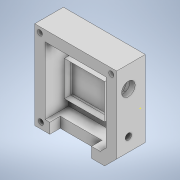
# Autodesk Inventor part: AmpClipOn
Saved by Autodesk Inventor 2020 (Build 240168000, 168)
## iProperties
Created: 2019-05-29
Part Number: AmpClipOn
Material: Generic
Document SubType Name: Modeling
Designer: Dammy
Density: 1 g/cm^3
Appearance: Default
Author: Dammy
Autodesk Inventor part; units mm, degrees
ref_plane "YZ Plane" through (0, 0, 0) normal (1, 0, 0) x (0, 1, 0)
ref_plane "XZ Plane" through (0, 0, 0) normal (0, 1, 0) x (-1, 0, 0)
ref_plane "XY Plane" through (0, 0, 0) normal (0, 0, 1) x (1, 0, 0)
sketch "Sketch1" plane through (0, 0, 0) normal (0, 0, 1) x (1, 0, 0)
  line L0 (11.825, -16.125) -> (-11.825, -16.125)
  line L1 (-14.625, -13.325) -> (-14.625, 16.125)
  line L2 (-14.625, 16.125) -> (14.625, 16.125)
  line L3 (14.625, 16.125) -> (14.625, -13.325)
  line L4 (14.625, -16.125) -> (-14.625, 16.125) construction
  line L5 (-14.625, -16.125) -> (14.625, 16.125) construction
  line L6 (11.825, -16.125) -> (14.625, -13.325)
  line L7 (-14.625, -13.325) -> (-14.625, -16.125)
  line L8 (-11.825, -16.125) -> (-14.625, -16.125)
  point P0 (0, 0)
  dimension "d0" = 29.25
  dimension "d1" = 32.25
  dimension "d56" = 2.8
  dimension "d57" = 2.8
  constraints: 18 end point, 4 point on line, 2 midpoint, 2 parallel, 2 perpendicular, 1 horizontal, 1 vertical
  measures "d0" distance of L1.end L2.end
  measures "d1" distance of L5.start L1.end
  measures "d56" distance of L0.start L4.start
  measures "d57" distance of L3.end L4.start
extrude "Extrusion1" add sketch "Sketch1" along normal blind 11.25
shell "Shell2" thickness 5 outward yes removed faces 1 at (-4.875, -3.5083, 11.25)
sketch "Sketch3" plane through (0, 0, 11.25) normal (0, 0, 1) x (1, 0, 0)
  line L0 (19.625, 21.125) -> (-19.625, 21.125) construction
  line L1 (-14.625, 16.125) -> (14.625, 16.125) construction
  line L2 (-19.625, 21.125) -> (-14.625, 16.125) construction
  line L3 (14.625, 16.125) -> (19.625, 21.125) construction
  line L4 (11.825, -16.125) -> (-14.625, -16.125) construction
  circle A0 centre (-17.125, 18.625) radius 1.25
  circle A1 centre (17.125, 18.625) radius 1.25
  line L5 (-14.625, -16.125) -> (-14.625, 16.125) construction
  line L6 (-14.625, -16.125) -> (-18.625, -20.125) construction
  circle A2 centre (-16.625, -18.125) radius 1.25
  point P0 (0, 0)
  point P1 (18.625, -20.125)
  point P2 (14.625, -16.125)
  point P3 (-11.825, -16.125)
  dimension "d14" = 2.5
  dimension "d15" = 2.5
  dimension "d58" = 2.5
  constraints: 6 end point, 3 centre point, 3 midpoint
  measures "d14" diameter of A0
  measures "d15" diameter of A1
  measures "d58" diameter of A2
extrude "Extrusion3" cut sketch "Sketch3" against normal through all
sketch "Sketch11" plane through (0, 0, 11.25) normal (0, 0, 1) x (1, 0, 0)
  line L0 (-19.625, -21.125) -> (13.8961, -21.125) projected
  line L1 (-14.625, -16.125) -> (11.825, -16.125) projected
  line L2 (7.625, -21.125) -> (-12.375, -21.125)
  line L3 (-12.375, -21.125) -> (-12.375, -16.125)
  line L4 (-12.375, -16.125) -> (7.625, -16.125)
  line L5 (7.625, -16.125) -> (7.625, -21.125)
  circle A0 centre (-16.625, -18.125) radius 1.25 projected
  line L6 (-19.625, 21.125) -> (-19.625, -21.125) projected
  point P0 (0, 0)
  point P1 (-13.4819, -20.125)
  point P2 (18.625, -20.125)
  point P3 (-11.825, -16.125)
  point P4 (14.625, -16.125)
  point P5 (13.8961, -21.125)
  point P6 (7.625, -16.125)
  dimension "d60" = 20
  dimension "d87" = 7.25
  constraints: 8 end point, 2 parallel, 1 horizontal, 1 perpendicular, 1 point on line, 2 other
  measures "d60" distance between parallel lines of L5 L3
  measures "d87" distance between parallel lines of L6 L3
extrude "Extrusion11" cut sketch "Sketch11" against normal blind 5 contours L3 L1 L5 L0
sketch "Sketch13" plane through (19.625, -15.3961, -5) normal (1, 0, 0) x (0, 0, -1)
  line L0 (-11.5, 18.8569) -> (-11.5, 3.8569) construction
  circle A0 centre (-10.625, 26.2711) radius 3.25
  line L1 (-16.25, 0) -> (-16.25, 36.5211) construction
  line L2 (0, 0) -> (-16.25, 0) construction
  line L3 (0, 36.5211) -> (-16.25, 36.5211) projected
  line L4 (-5, 2.0711) -> (-5, 31.5211) projected
  point P0 (-5, 15.3961)
  dimension "d61" = 6.5
  dimension "d81" = 10.25
  dimension "d86" = 5.625
  constraints: 1 centre point
  measures "d61" diameter of A0
  measures "d81" distance from line of L3 A0.centre
  measures "d86" distance from line of A0.centre L4
extrude "Extrusion13" cut sketch "Sketch13" against normal up to surface (5 mm away)
sketch "Sketch14" plane through (-14.625, 16.125, 0) normal (0, 0, 1) x (1, 0, 0)
  line L0 (2, -11.5) -> (19.25, -11.5)
  line L1 (19.25, -11.5) -> (19.25, -26.25)
  line L2 (19.25, -26.25) -> (2, -26.25)
  line L3 (2, -26.25) -> (2, -11.5)
  line L4 (1.25, -10.5) -> (20, -10.5)
  line L5 (20.25, -11.25) -> (20.25, -27)
  line L6 (19.45, -27.25) -> (1.25, -27.25)
  line L7 (1, -27) -> (1, -10.75)
  line L8 (0, -32.25) -> (0, 0) projected
  line L9 (2.25, -32.25) -> (0, -32.25) projected
  line L10 (20, -10.5) -> (20.25, -10.5)
  line L11 (20.25, -10.5) -> (20.25, -11.25)
  line L12 (19.45, -27.25) -> (20.25, -27.25)
  line L13 (20.25, -27.25) -> (20.25, -27)
  line L14 (1.25, -27.25) -> (1, -27.25)
  line L15 (1, -27) -> (1, -27.25)
  line L16 (1, -10.75) -> (1, -10.5)
  line L17 (1.25, -10.5) -> (1, -10.5)
  point P0 (14.625, -16.125)
  point P1 (10.625, -11.5)
  point P2 (10.625, -10.5)
  point P3 (1, -18.875)
  point P4 (2, -18.875)
  dimension "d66" = 1
  dimension "d67" = 1
  dimension "d69" = 17.25
  dimension "d70" = 14.75
  dimension "d71" = 1
  dimension "d72" = 5
  dimension "d83" = 1
  dimension "d84" = 1
  constraints: 32 end point, 7 perpendicular, 5 point on line, 4 midpoint, 4 parallel, 3 horizontal, 1 horizontal alignment, 1 vertical alignment
  measures "d66" distance between parallel lines of L4 L0
  measures "d67" distance between parallel lines of L3 L7
  measures "d69" distance of L0.start L0.end
  measures "d70" distance between parallel lines of L0 L2
  measures "d71" distance between parallel lines of L8 L7
  measures "d72" distance between parallel lines of L9 L6
  measures "d83" distance between parallel lines of L1 L5
  measures "d84" distance between parallel lines of L2 L6
extrude "Extrusion14" add sketch "Sketch14" along normal blind 3
sketch "Sketch15" plane through (0, 0, -5) normal (0, 0, -1) x (-1, 0, 0)
  line L0 (-19.625, -15.3961) -> (-19.625, 21.125) projected
  line L1 (19.625, -21.125) -> (-13.8961, -21.125) projected
  line L2 (-19.625, 21.125) -> (19.625, 21.125)
  line L3 (19.625, 21.125) -> (19.625, -21.125)
  line L4 (19.625, -21.125) -> (-19.625, -21.125)
  line L5 (-19.625, -21.125) -> (-19.625, 21.125)
  point P0 (0, 0)
  constraints: 8 end point, 2 parallel, 1 horizontal, 1 perpendicular
extrude "Extrusion15" cut sketch "Sketch15" against normal blind 2.5
sketch "Sketch16" plane through (19.625, -15.3961, 11.25) normal (1, 0, 0) x (0, 0, -1)
  point P0 (11.25, 15.3961)
sketch "Sketch17" plane through (19.625, -15.3961, 11.25) normal (1, 0, 0) x (0, 0, -1)
  circle A0 centre (5.625, 6.5) radius 1.5
  circle A1 centre (5.625, 26.2711) radius 3.25 projected
  line L0 (13.75, 0) -> (0, 0) projected
  point P0 (11.25, 15.3961)
  point P1 (0.8377, 31.1069)
  point P2 (7.1623, 31.1069)
  dimension "d77" = 3
  dimension "d82" = 6.5
  constraints: 1 centre point, 1 coincident, 1 vertical alignment, 1 other
  measures "d77" diameter of A0
  measures "d82" distance from line of L0 A0.centre
extrude "Extrusion16" cut sketch "Sketch17" against normal up to surface (5 mm away) contours A0
fillet "Fillet1" radius 2.5 4 edges at (-4, 4.625, 3) (-12.625, -2.75, 3) (-4, -10.125, 3) (4.625, -2.75, 3)
sketch "Sketch18" plane through (14.625, -13.325, 0) normal (-1, 0, 0) x (0, 0, 1)
  circle A0 centre (5.625, 24.2) radius 3.25 construction
  circle A1 centre (5.625, 24.2) radius 4.6 construction
  line L0 (7.0969, 28.8) -> (11.5207, 28.8) construction
  line L1 (5.625, 28.8) -> (5.625, 19.6) construction
  line L2 (1.025, 24.2) -> (10.225, 24.2) construction
  line L3 (5.625, 24.2) -> (10.225, 24.2) construction
  line L4 (10.225, 24.2) -> (11.25, 24.2) construction
  line L5 (11.25, 29.45) -> (11.25, 0) construction
  line L6 (8.2808, 28.8) -> (10.9366, 24.2)
  line L7 (10.9366, 24.2) -> (8.2808, 19.6)
  line L8 (8.2808, 19.6) -> (2.9692, 19.6)
  line L9 (2.9692, 19.6) -> (0.3134, 24.2)
  line L10 (0.3134, 24.2) -> (2.9692, 28.8)
  line L11 (2.9692, 28.8) -> (8.2808, 28.8)
  point P0 (0, 13.325)
  point P1 (9.1346, 27.1737)
  dimension "d88" = 9.2
  constraints: 22 end point, 5 point on circle, 3 horizontal, 2 coincident, 2 midpoint, 1 centre point, 1 horizontal alignment, 1 perpendicular, 1 point on line, 1 vertical, 13 other
  measures "d88" diameter of A1
extrude "Extrusion17" cut sketch "Sketch18" against normal blind 2.5
equation "\"d57\" = d56"
equation "\"d58\" = d14"
equation "\"d86\" = 0.5 * d4"
equation "\"d71\" = d67"
equation "\"d83\" = d67"
equation "\"d84\" = d67"
equation "\"d92\" = 0.5 * d13"
equation "\"d4\" = 11.25"
equation "\"d13\" = 5"
body "Solid1"
